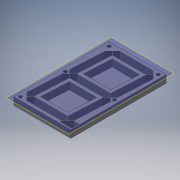
# Autodesk Inventor part: Segment_V2
Saved by Autodesk Inventor 2016 SP2 (Build 200236200, 236)
## iProperties
Created: 2018-06-10
Part Number: Segment_V2
Material: Generisch
Document SubType Name: Modeling
Designer: Nils
Density: 1 g/cm^3
Appearance: Vorgabe
Author: Nils
Autodesk Inventor part; units mm, degrees
ref_plane "YZ Plane" through (0, 0, 0) normal (1, 0, 0) x (0, 1, 0)
ref_plane "XZ Plane" through (0, 0, 0) normal (0, 1, 0) x (-1, 0, 0)
ref_plane "XY Plane" through (0, 0, 0) normal (0, 0, 1) x (1, 0, 0)
ref_plane "Arbeitsebene1" through (-207.5632, -47.4012, -6.8891) normal (0, 0, -1) x (-1, 0, 0)
sketch "Skizze1" plane through (-207.5632, -47.4012, -6.8891) normal (0, 0, -1) x (-1, 0, 0)
  line L0 (-22.8942, -55.5591) -> (-25.5022, -5.7954) projected
  line L1 (-25.5022, -5.7954) -> (-30.8485, -0.4491) projected
  line L2 (-30.8485, -0.4491) -> (-35.9303, -5.5309) projected
  line L3 (-35.9303, -5.5309) -> (-33.2659, -56.3721) projected
  line L4 (-33.2659, -56.3721) -> (-32.7821, -56.3468) projected
  line L5 (-32.7821, -56.3468) -> (-28.232, -60.8969) projected
  line L6 (-22.8942, -55.5591) -> (-28.232, -60.8969) projected
  line L7 (-27.6418, -61.4871) -> (-22.5832, -66.5457) projected
  line L8 (-22.5832, -66.5457) -> (27.8168, -66.5457) projected
  line L9 (27.8168, -66.5457) -> (32.8754, -61.4871) projected
  line L10 (27.534, -56.1457) -> (32.8754, -61.4871) projected
  line L11 (27.534, -56.1457) -> (-22.3004, -56.1457) projected
  line L12 (-27.6418, -61.4871) -> (-22.3004, -56.1457) projected
  line L13 (-33.4653, 60.8966) -> (-28.119, 55.5503) projected
  line L14 (-33.4653, 60.8966) -> (-38.5471, 55.8148) projected
  line L15 (-38.5471, 55.8148) -> (-35.8827, 4.9736) projected
  line L16 (-35.8827, 4.9736) -> (-35.3984, 4.9989) projected
  line L17 (-35.3984, 4.9989) -> (-30.8485, 0.4491) projected
  line L18 (-30.8485, 0.4491) -> (-25.511, 5.7866) projected
  line L19 (-25.511, 5.7866) -> (-28.119, 55.5503) projected
  circle A0 centre (-36.6168, 0) radius 2.5 projected
  circle A1 centre (-36.6168, 65.3457) radius 2.5 projected
  circle A2 centre (36.6168, 65.3457) radius 2.5 projected
  circle A3 centre (36.6168, 0) radius 2.5 projected
  circle A4 centre (37.6168, -66.3457) radius 2.5 projected
  line L20 (-32.9803, -57.8457) -> (-41.4168, -57.8457) projected
  line L21 (-41.4168, -57.8457) -> (-41.4168, -68.8457) projected
  line L22 (-41.4168, -68.8457) -> (-24.4168, -68.8457) projected
  line L23 (-24.4168, -68.8457) -> (-24.4168, -66.4092) projected
  line L24 (-24.4168, -66.4092) -> (-32.9803, -57.8457) projected
  line L25 (42.6168, 71.3457) -> (42.6168, -71.3457) projected
  line L26 (42.6168, -71.3457) -> (-42.6168, -71.3457) projected
  line L27 (-42.6168, -71.3457) -> (-42.6168, 71.3457) projected
  line L28 (-42.6168, 71.3457) -> (42.6168, 71.3457) projected
  line L29 (22.8813, -51.1457) -> (20.7354, -10.2) projected
  line L30 (20.7354, -10.2) -> (-20.2645, -10.2) projected
  line L31 (-20.2645, -10.2) -> (-18.1186, -51.1457) projected
  line L32 (-18.1186, -51.1457) -> (22.8813, -51.1457) projected
  line L33 (18.1186, 51.1457) -> (-22.8813, 51.1457) projected
  line L34 (-22.8813, 51.1457) -> (-20.7354, 10.2) projected
  line L35 (-20.7354, 10.2) -> (20.2645, 10.2) projected
  line L36 (20.2645, 10.2) -> (18.1186, 51.1457) projected
  line L37 (22.3004, 56.1457) -> (27.6418, 61.4871) projected
  line L38 (27.6418, 61.4871) -> (22.5832, 66.5457) projected
  line L39 (22.5832, 66.5457) -> (-27.8168, 66.5457) projected
  line L40 (-27.8168, 66.5457) -> (-32.8754, 61.4871) projected
  line L41 (-27.534, 56.1457) -> (-32.8754, 61.4871) projected
  line L42 (-27.534, 56.1457) -> (22.3004, 56.1457) projected
  line L43 (33.4653, -60.8966) -> (28.119, -55.5503) projected
  line L44 (33.4653, -60.8966) -> (38.5471, -55.8148) projected
  line L45 (38.5471, -55.8148) -> (35.8827, -4.9736) projected
  line L46 (35.8827, -4.9736) -> (35.3984, -4.9989) projected
  line L47 (35.3984, -4.9989) -> (30.8485, -0.4491) projected
  line L48 (30.8485, -0.4491) -> (25.511, -5.7866) projected
  line L49 (25.511, -5.7866) -> (28.119, -55.5503) projected
  line L50 (30.8488, 0.4488) -> (35.9439, 5.5439) projected
  line L51 (35.9439, 5.5439) -> (33.2801, 56.3729) projected
  line L52 (33.2801, 56.3729) -> (32.7816, 56.3468) projected
  line L53 (32.7816, 56.3468) -> (28.2317, 60.8966) projected
  line L54 (28.2317, 60.8966) -> (22.8942, 55.5591) projected
  line L55 (22.8942, 55.5591) -> (25.5022, 5.7954) projected
  line L56 (25.5022, 5.7954) -> (30.8488, 0.4488) projected
  line L57 (24.9172, -5.2) -> (30.1172, 0) projected
  line L58 (30.1172, 0) -> (24.9172, 5.2) projected
  line L59 (24.9172, 5.2) -> (-24.9172, 5.2) projected
  line L60 (-24.9172, 5.2) -> (-30.1172, 0) projected
  line L61 (-30.1172, 0) -> (-24.9172, -5.2) projected
  line L62 (-24.9172, -5.2) -> (24.9172, -5.2) projected
  point P0 (-207.5632, 47.4012)
extrude "Extrusion1" add sketch "Skizze1" along normal blind 10.5 contours A0 | A1 | A2 | A3 | A4 | L25 L26 L27 L28
sketch "Skizze2" plane through (-207.5632, -47.4012, -17.3891) normal (0, 0, -1) x (-1, 0, 0)
  line L0 (42.6168, 71.3457) -> (-42.6168, 71.3457) projected
  line L1 (-42.6168, 71.3457) -> (-42.6168, -71.3457) projected
  line L2 (42.6168, -71.3457) -> (42.6168, 71.3457) projected
  line L3 (-42.6168, -71.3457) -> (42.6168, -71.3457) projected
  circle A0 centre (-21.5004, -57.8457) radius 1.75
  circle A1 centre (26.734, -57.8457) radius 1.75
  circle A2 centre (-39.7168, -67.1457) radius 1.75
  circle A3 centre (-26.1168, -67.1457) radius 1.75
  circle A4 centre (-24.6385, -54.7591) radius 1.75
  circle A5 centre (29.7794, -54.7503) radius 1.75
  circle A6 centre (27.2553, -6.5866) radius 1.75
  circle A7 centre (-27.1626, -6.5954) radius 1.75
  circle A8 centre (-24.1172, -3.5) radius 1.75
  circle A9 centre (24.1172, -3.5) radius 1.75
  circle A10 centre (-27.2553, 6.5866) radius 1.75
  circle A11 centre (27.1626, 6.5954) radius 1.75
  circle A12 centre (-29.7794, 54.7503) radius 1.75
  circle A13 centre (24.6385, 54.7591) radius 1.75
  circle A14 centre (21.5004, 57.8457) radius 1.75
  circle A15 centre (-26.734, 57.8457) radius 1.75
  line L4 (25.5022, 5.7954) -> (22.8942, 55.5591) projected
  line L5 (22.3004, 56.1457) -> (-27.534, 56.1457) projected
  line L6 (-25.511, 5.7866) -> (-28.119, 55.5503) projected
  line L7 (24.9172, -5.2) -> (-24.9172, -5.2) projected
  line L8 (-22.8942, -55.5591) -> (-25.5022, -5.7954) projected
  line L9 (28.119, -55.5503) -> (25.511, -5.7866) projected
  line L10 (-22.3004, -56.1457) -> (27.534, -56.1457) projected
  line L11 (-24.4168, -68.8457) -> (-41.4168, -68.8457) projected
  line L12 (-24.4168, -66.4092) -> (-24.4168, -68.8457) projected
  line L13 (-41.4168, -68.8457) -> (-41.4168, -57.8457) projected
  point P0 (-207.5632, 47.4012)
  dimension "d2" = 3.5
  dimension "d3" = 3.5
  dimension "d4" = 3.5
  dimension "d5" = 3.5
  dimension "d6" = 3.5
  dimension "d7" = 3.5
  dimension "d8" = 3.5
  dimension "d9" = 3.5
  dimension "d10" = 3.5
  dimension "d11" = 3.5
  dimension "d12" = 3.5
  dimension "d13" = 3.5
  dimension "d14" = 3.5
  dimension "d15" = 3.5
  dimension "d16" = 3.5
  dimension "d17" = 3.5
  dimension "d18" = 1.7
  dimension "d19" = 1.7
  dimension "d20" = 1.7
  dimension "d21" = 1.7
  dimension "d22" = 1.7
  dimension "d23" = 1.7
  dimension "d24" = 1.7
  dimension "d25" = 1.7
  dimension "d26" = 1.7
  dimension "d27" = 1.7
  dimension "d28" = 1.7
  dimension "d29" = 1.7
  dimension "d30" = 1.7
  dimension "d31" = 1.7
  dimension "d32" = 1.7
  dimension "d33" = 1.7
  dimension "d34" = 1.7
  dimension "d35" = 1.7
  dimension "d36" = 0.8
  dimension "d37" = 0.8
  dimension "d38" = 0.8
  dimension "d39" = 0.8
  dimension "d40" = 0.8
  dimension "d41" = 0.8
  dimension "d42" = 0.8
  dimension "d43" = 0.8
  dimension "d44" = 0.8
  dimension "d45" = 0.8
  dimension "d46" = 0.8
  dimension "d47" = 0.8
  dimension "d48" = 0.8
  dimension "d49" = 0.8
  constraints: 16 centre point
  measures "d2" diameter of A0
  measures "d3" diameter of A3
  measures "d4" diameter of A2
  measures "d5" diameter of A4
  measures "d6" diameter of A1
  measures "d7" diameter of A5
  measures "d8" diameter of A6
  measures "d9" diameter of A9
  measures "d10" diameter of A8
  measures "d11" diameter of A7
  measures "d12" diameter of A10
  measures "d13" diameter of A11
  measures "d14" diameter of A12
  measures "d15" diameter of A15
  measures "d16" diameter of A14
  measures "d17" diameter of A13
  measures "d18" distance from line of L4 A13.centre
  measures "d19" distance from line of A14.centre L5
  measures "d20" distance from line of L5 A15.centre
  measures "d21" distance from line of L6 A12.centre
  measures "d22" distance from line of L6 A10.centre
  measures "d23" distance from line of L4 A11.centre
  measures "d24" distance from line of L7 A9.centre
  measures "d25" distance from line of L7 A8.centre
  measures "d26" distance from line of L8 A7.centre
  measures "d27" distance from line of L9 A6.centre
  measures "d28" distance from line of L9 A5.centre
  measures "d29" distance from line of L10 A1.centre
  measures "d30" distance from line of L10 A0.centre
  measures "d31" distance from line of L11 A3.centre
  measures "d32" distance from line of L11 A2.centre
  measures "d33" distance from line of L8 A4.centre
  measures "d34" distance from line of L12 A3.centre
  measures "d35" distance from line of L13 A2.centre
  measures "d36" horizontal distance of L10.end A1.centre
  measures "d37" horizontal distance of A0.centre L10.start
  measures "d38" vertical distance of L8.start A4.centre
  measures "d39" vertical distance of L8.end A7.centre
  measures "d40" horizontal distance of L7.end A8.centre
  measures "d41" horizontal distance of L7.start A9.centre
  measures "d42" vertical distance of L9.end A6.centre
  measures "d43" vertical distance of L4.start A11.centre
  measures "d44" vertical distance of A13.centre L4.end
  measures "d45" horizontal distance of L5.start A14.centre
  measures "d46" horizontal distance of L5.end A15.centre
  measures "d47" vertical distance of L6.end A12.centre
  measures "d48" vertical distance of L6.start A10.centre
  measures "d49" vertical distance of L9.start A5.centre
extrude "Extrusion2" add sketch "Skizze2" along normal blind 0.8 contours L2 L3 L1 L0 | A2 L11 L13 | A3 L12 L11 picked at (-41.1035, -68.5324) picked at (-24.7301, -68.5324)
sketch "Skizze3" plane through (-207.5632, -47.4012, -6.8891) normal (0, 0, 1) x (1, 0, 0)
  circle A0 centre (-37.6168, -66.3457) radius 2.5 projected
  circle A1 centre (36.6168, 0) radius 2.5 projected
  circle A2 centre (-36.6168, 0) radius 2.5 projected
  circle A3 centre (-36.6168, 65.3457) radius 2.5 projected
  circle A4 centre (36.6168, 65.3457) radius 2.5 projected
  point P0 (207.5632, 47.4012)
extrude "Extrusion3" cut sketch "Skizze3" against normal blind 3
sketch "Skizze4" plane through (-207.5632, -47.4012, -18.1891) normal (0, 0, -1) x (-1, 0, 0)
  circle A0 centre (-36.6168, 0) radius 2.5 projected
  circle A1 centre (37.6168, -66.3457) radius 2.5 projected
  circle A2 centre (36.6168, 0) radius 2.5 projected
  circle A3 centre (36.6168, 65.3457) radius 2.5 projected
  circle A4 centre (-36.6168, 65.3457) radius 2.5 projected
  point P0 (-207.5632, 47.4012)
extrude "Extrusion4" cut sketch "Skizze4" against normal blind 3
equation "\"d3\" = d2"
equation "\"d4\" = d2"
equation "\"d5\" = d2"
equation "\"d6\" = d2"
equation "\"d7\" = d2"
equation "\"d8\" = d2"
equation "\"d9\" = d2"
equation "\"d10\" = d2"
equation "\"d11\" = d2"
equation "\"d12\" = d2"
equation "\"d13\" = d2"
equation "\"d14\" = d2"
equation "\"d15\" = d2"
equation "\"d16\" = d2"
equation "\"d17\" = d2"
equation "\"d19\" = d18"
equation "\"d20\" = d18"
equation "\"d21\" = d18"
equation "\"d22\" = d18"
equation "\"d23\" = d18"
equation "\"d24\" = d18"
equation "\"d25\" = d18"
equation "\"d26\" = d18"
equation "\"d27\" = d18"
equation "\"d28\" = d18"
equation "\"d29\" = d18"
equation "\"d30\" = d18"
equation "\"d31\" = d18"
equation "\"d32\" = d18"
equation "\"d33\" = d18"
equation "\"d34\" = d18"
equation "\"d35\" = d18"
equation "\"d37\" = d36"
equation "\"d38\" = d36"
equation "\"d39\" = d36"
equation "\"d40\" = d36"
equation "\"d41\" = d36"
equation "\"d42\" = d36"
equation "\"d43\" = d36"
equation "\"d44\" = d36"
equation "\"d45\" = d36"
equation "\"d46\" = d36"
equation "\"d47\" = d36"
equation "\"d48\" = d36"
equation "\"d49\" = d36"
